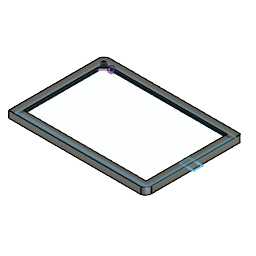
vwr_96_wp_deck_i2 (Autodesk Fusion 360 design; units mm, degrees)
part number: 2026-04-28-02-08-20-957
Autodesk Fusion 360 part; units mm, degrees
sketch "Sketch1" plane through (0, 0, 0) normal (0, 0, 1) x (1, 0, 0)
  line L0 (-64, 43.05) -> (64, 43.05)
  line L1 (64, 43.05) -> (64, -43.05)
  line L2 (64, -43.05) -> (-64, -43.05)
  line L3 (-64, -43.05) -> (-64, 43.05)
  line L4 (0, 43.05) -> (0, -43.05)
  dimension "d5" = 128
  dimension "d6" = 86.1
  constraint horizontal L0
  constraint vertical L1
  constraint horizontal L2
  constraint vertical L3
  constraint midpoint L0 L4.start
  constraint midpoint L2 L4.end
  constraint midpoint origin L4
  measures "d5" distance of L0.start L0.end
  measures "d6" distance of L0.start L2.end
extrude "Extrude1" add sketch "Sketch1" along normal blind 3 makes body 1
fillet "Fillet1" radius 1 4 edges at (64, 43.05, 1.5) (-64, 43.05, 1.5) (-64, -43.05, 1.5) (64, -43.05, 1.5) on bodies 1
sketch "Sketch2" plane through (0, 0, 3) normal (0, 0, 1) x (-1, 0, 0)
  arc A0 (-63, 43.05) -> (-64, 42.05) centre (-63, 42.05) ccw
  line L0 (-64, 42.05) -> (-64, -42.05)
  arc A1 (-64, -42.05) -> (-63, -43.05) centre (-63, -42.05) ccw
  line L1 (-63, -43.05) -> (63, -43.05)
  arc A2 (63, -43.05) -> (64, -42.05) centre (63, -42.05) ccw
  line L2 (64, -42.05) -> (64, 42.05)
  arc A3 (64, 42.05) -> (63, 43.05) centre (63, 42.05) ccw
  line L3 (63, 43.05) -> (-63, 43.05)
  line L4 (-10.1311, 43.05) -> (-10.1311, 40.45)
  line L5 (64, 40.7331) -> (61.4, 40.7331)
  line L6 (61.4, 40.7331) -> (-62.6, 40.7331)
  line L7 (-62.6, 40.7331) -> (-62.6, -41.3669)
  line L8 (-62.6, -41.3669) -> (61.4, -41.3669)
  line L9 (61.4, -41.3669) -> (61.4, 40.7331)
  dimension "d12" = 2.6
  dimension "d13" = 2.6
  dimension "d16" = 124
  dimension "d17" = 82.1
  constraint coincident L3 L4.start
  constraint perpendicular L3 L4
  constraint coincident L2 L5.start
  constraint perpendicular L2 L5
  constraint horizontal L6
  constraint vertical L7
  constraint horizontal L8
  constraint vertical L9
  measures "d12" distance of L4.start L4.end
  measures "d13" distance of L5.start L5.end
extrude "Extrude2" add sketch "Sketch2" along normal blind 12.1 contours L6 L7 L8 L9 bodies 1
chamfer "Chamfer1" distance 6.8 angle 45 1 edges at (-61.4, 41.3669, 9.05) on bodies 1
sketch "Sketch3" plane through (0, 0, 3) normal (0, 0, 1) x (-1, 0, 0)
  line L0 (54.6, -41.3669) -> (-62.6, -41.3669)
  line L1 (-62.6, -41.3669) -> (-62.6, 40.7331)
  line L2 (-62.6, 40.7331) -> (61.4, 40.7331)
  line L3 (61.4, 40.7331) -> (61.4, -34.5669)
  arc A0 (-63, 43.05) -> (-64, 42.05) centre (-63, 42.05) ccw
  line L4 (-64, 42.05) -> (-64, -42.05)
  arc A1 (-64, -42.05) -> (-63, -43.05) centre (-63, -42.05) ccw
  line L5 (-63, -43.05) -> (63, -43.05)
  arc A2 (63, -43.05) -> (64, -42.05) centre (63, -42.05) ccw
  line L6 (64, -42.05) -> (64, 42.05)
  arc A3 (64, 42.05) -> (63, 43.05) centre (63, 42.05) ccw
  line L7 (63, 43.05) -> (-63, 43.05)
  line L8 (63.7071, 42.7571) -> (-64.2929, 42.7571)
  line L9 (-64.2929, 42.7571) -> (-64.2929, -43.7218)
  line L10 (-64.2929, -43.7218) -> (63.7071, -43.3429)
  line L11 (63.7071, -43.3429) -> (63.7071, 42.7571)
  line L12 (61.4, -34.5669) -> (54.6, -41.3669)
  dimension "d22" = 128
  dimension "d23" = 86.1
  constraint horizontal L8
  constraint vertical L9
  constraint vertical L11
  constraint midpoint A3 L8.start
  measures "d22" distance of L8.start L8.end
  measures "d23" distance of L8.start L10.end
extrude "Extrude3" add sketch "Sketch3" along normal blind 2 separate body contours A0 L4 A1 L5 A2 L8 L11 makes body 2
move_face "OffsetFaces1" offset 5.5 4 faces at (64, -14.0167, 3.6667) (21.2357, -42.7571, 4.3333) (-63.7071, 14.2524, 3.6667) (21, 43.05, 3.6667) on bodies 2
sketch "Sketch4" plane through (0, 0, 3) normal (0, 0, -1) x (1, 0, 0)
  arc A0 (68.5, -48.55) -> (69.5, -47.55) centre (68.5, -47.55) ccw
  line L0 (69.5, -47.55) -> (69.5, 42.05)
  arc A1 (69.5, 42.05) -> (64.9292, 48.2571) centre (63, 42.05) ccw
  line L1 (64.9292, 48.2571) -> (-69.2071, 48.2571)
  line L2 (-69.2071, 48.2571) -> (-69.2071, -43.9792)
  arc A2 (-69.2071, -43.9792) -> (-63, -48.55) centre (-63, -42.05) ccw
  line L3 (-63, -48.55) -> (68.5, -48.55)
  line L4 (62.6, -41.3669) -> (-54.6, -41.3669)
  line L5 (-61.4, -34.5669) -> (-61.4, 40.7331)
  line L6 (-61.4, 40.7331) -> (62.6, 40.7331)
  line L7 (62.6, 40.7331) -> (62.6, -41.3669)
  line L8 (67.2117, 44.8466) -> (-65.3311, 44.8466)
  line L9 (-65.3311, 44.8466) -> (-65.3311, -45.1406)
  line L10 (-65.3311, -45.1406) -> (67.2117, -45.1406)
  line L11 (67.2117, -45.1406) -> (67.2117, 44.8466)
  line L12 (65.8712, 43.05) -> (-63, 43.05)
  line L13 (-63, 43.05) -> (-63, -42.05)
  line L14 (-63, -42.05) -> (65.8712, -42.05)
  line L15 (65.8712, -42.05) -> (65.8712, 43.05)
  line L16 (75.9734, 5.7216) -> (61.8734, 5.7216)
  line L17 (61.8734, 5.7216) -> (61.8734, -3.2784)
  line L18 (61.8734, -3.2784) -> (75.9734, -3.2784)
  line L19 (75.9734, -3.2784) -> (75.9734, 5.7216)
  line L20 (-54.6, -41.3669) -> (-61.4, -34.5669)
  dimension "d62" = 14.1
  dimension "d63" = 9
  constraint horizontal L8
  constraint vertical L9
  constraint horizontal L10
  constraint vertical L11
  constraint horizontal L12
  constraint vertical L13
  constraint horizontal L14
  constraint vertical L15
  constraint coincident A2.centre L13.end
  constraint horizontal L16
  constraint vertical L17
  constraint horizontal L18
  constraint vertical L19
  measures "d62" distance of L16.start L16.end
  measures "d63" distance of L16.start L18.end
extrude "Extrude6" add sketch "Sketch4" along normal blind 5 contours A0 L0 A1 L1 L2 A2 L3 L8 L9 L10 L11 L16 L18 | L0 L11 L16 L18 bodies 2
extrude "Extrude7" add sketch "Sketch4" along normal blind 5 contours A0 L0 A1 L1 L2 A2 L3 L8 L9 L10 L11 L16 L18 | L0 L11 L16 L18 bodies 2
extrude "Extrude8" add sketch "Sketch4" along normal blind 1 contours L11 L15 L16 L18 | L8 L9 L10 L11 L12 L13 L14 L15 L16 L18 bodies 2
hidden bodies 1
equation "width = 128 mm"
equation "length = 86.1 mm"
equation "base_h = 3.1 mm"
equation "platform_h = 14.1 mm"
equation "d5 = width"
equation "d6 = length"
equation "d7 = top_piece_h"
equation "base_platform_gap = 2.6 mm"
equation "d12 = base_platform_gap"
equation "d13 = base_platform_gap"
equation "platform_width = width - 4 mm"
equation "platform_length = length - 4 mm"
equation "d16 = platform_width"
equation "d17 = platform_length"
equation "platform_shell_depth = 6.8 mm"
equation "d21 = platform_shell_depth"
equation "d22 = width"
equation "d23 = length"
equation "deck_platform_cover_height = 2 mm"
equation "d25 = deck_platform_cover_height"
equation "d27 = deck_base_cover_distance"
equation "deck_base_cover_distance = 5.5 mm"
equation "dmag_6mm = 6.4 mm"
equation "dmag_8mm = 8.4 mm"
equation "dmag_10mm = 10.4 mm"
equation "dmag_thickness = 2.2 mm"
equation "plate_base__depth = 3.3 mm"
equation "top_piece_h = 3 mm"
equation "base_w = 90 mm"
equation "base_l = 131.5 mm"
equation "d47 = base_deck_depth"
equation "weight_incision_l_width = 22 mm"
equation "weight_incision_l_length = 130 mm"
equation "base_deck_depth = 5 mm"
equation "d54 = base_deck_depth"
equation "filling_h = 1 mm"
equation "d57 = filling_h"
equation "clamp_w = 14.1 mm"
equation "clamp_l = 9 mm"
equation "clamp_thickness = 7 mm"
equation "d62 = clamp_w"
equation "d63 = clamp_l"
named bodies: "96wellplate", "deck"
